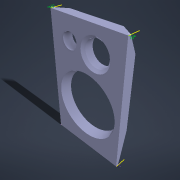
# Autodesk Inventor part: Front
Saved by Autodesk Inventor 2022 (Build 260153000, 153)
## iProperties
Created: 2022-03-29
Part Number: Front
Material: Пластик АБС
Document SubType Name: Modeling
Designer: Kalugin_a
Density: 1.06 g/cm^3
Appearance: Грифельно-синий
Author: Kalugin_a
Autodesk Inventor part; units mm, degrees
ref_plane "YZ Plane" through (0, 0, 0) normal (1, 0, 0) x (0, 1, 0)
ref_plane "XZ Plane" through (0, 0, 0) normal (0, 1, 0) x (-1, 0, 0)
ref_plane "XY Plane" through (0, 0, 0) normal (0, 0, 1) x (1, 0, 0)
sketch "Эскиз1" plane through (0, 0, 0) normal (0, 0, 1) x (1, 0, 0)
  line L0 (0, 0) -> (290, 0)
  line L1 (290, 0) -> (290, 470)
  line L2 (290, 470) -> (0, 470)
  line L3 (0, 470) -> (0, 0)
  line L4 (145, 470) -> (145, 0) construction
  circle A0 centre (145, 180) radius 133
  circle A1 centre (145, 180) radius 115
  circle A2 centre (80, 390) radius 47
  circle A3 centre (80, 390) radius 30
  line L5 (136.9264, 433.5) -> (229.9264, 433.5)
  line L6 (236.9264, 426.5) -> (236.9264, 333.5)
  line L7 (229.9264, 326.5) -> (136.9264, 326.5)
  line L8 (129.9264, 333.5) -> (129.9264, 426.5)
  line L9 (129.9264, 433.5) -> (236.9264, 326.5) construction
  line L10 (236.9264, 433.5) -> (129.9264, 326.5) construction
  circle A4 centre (183.4264, 380) radius 47
  circle A5 centre (183.4264, 380) radius 58 construction
  line L11 (0, 160) -> (60, 0)
  line L12 (290, 160) -> (230, 0)
  line L13 (50, 470) -> (0, 400)
  line L14 (240, 470) -> (290, 400)
  line L15 (290, 320) -> (0, 320) construction
  arc A6 (236.9264, 429.5) -> (232.9264, 433.5) centre (232.9264, 429.5) ccw
  arc A7 (236.9264, 426.5) -> (229.9264, 433.5) centre (229.9264, 426.5) ccw
  arc A8 (136.9264, 433.5) -> (129.9264, 426.5) centre (136.9264, 426.5) ccw
  arc A9 (129.9264, 333.5) -> (136.9264, 326.5) centre (136.9264, 333.5) ccw
  arc A10 (229.9264, 326.5) -> (236.9264, 333.5) centre (229.9264, 333.5) ccw
  line L16 (0, 320) -> (290, 320)
  dimension "d0" = 290
  dimension "d1" = 470
  dimension "d3" = 266
  dimension "d4" = 230
  dimension "d5" = 94
  dimension "d6" = 60
  dimension "d9" = 94
  dimension "d11" = 380
  dimension "d12" = 390
  dimension "d13" = 180
  dimension "d14" = 160
  dimension "d15" = 60
  dimension "d16" = 160
  dimension "d17" = 60
  dimension "d18" = 50
  dimension "d19" = 70
  dimension "d20" = 80
  dimension "d21" = 50
  dimension "d38" = 70
  dimension "d39" = 320
  dimension "d47" = 4
  dimension "d48" = 7
  constraints: 34 end point, 20 point on line, 11 centre point, 10 point on circle, 10 tangent, 5 equal length, 4 perpendicular, 3 coincident, 3 equal radius, 3 horizontal, 3 midpoint
  measures "d0" distance of L2.end L1.end
  measures "d1" distance of L1.end L0.end
  measures "d3" diameter of A0
  measures "d4" diameter of A1
  measures "d5" diameter of A2
  measures "d6" diameter of A3
  measures "d9" diameter of A4
  measures "d11" distance from line of L0 A5.centre
  measures "d12" distance from line of L0 A2.centre
  measures "d13" distance of L4.end A0.centre
  measures "d14" distance of L0.start L11.start
  measures "d15" distance of L0.start L11.end
  measures "d16" distance of L0.end L12.start
  measures "d17" distance of L0.end L12.end
  measures "d18" distance of L2.end L13.start
  measures "d19" distance of L2.end L13.end
  measures "d20" distance from line of L3 A2.centre
  measures "d21" distance of L1.end L14.start
  measures "d38" distance of L1.end L14.end
  measures "d39" distance between parallel lines of L0 L15
  measures "d47" radius of A6
  measures "d48" radius of A7
extrude "Выдавливание1" add sketch "Эскиз1" along normal blind 42 contours L3 L11 L0 | L11 L3 L16 L1 L12 L0 | L12 L1 L0 | L3 L13 L2 L14 L1 L16 | L3 L2 L13 | L14 L2 L1 | A0 | A2 | L5 A7 L6 A10 L7 A9 L8 A8
sketch "Эскиз3" plane through (0, 470, 0) normal (0, 1, 0) x (1, 0, 0)
  line L0 (290, 0) -> (290, -42) projected
  line L1 (0, 0) -> (0, -42) projected
  point P0 (290, -32)
  point P1 (0, -32)
  dimension "d24" = 10
  dimension "d25" = 10
  constraints: 2 point on line
  measures "d24" distance of L0.end point (290, -32)
  measures "d25" distance of L1.end point (0, -32)
sketch "Эскиз4" plane through (0, 0, 0) normal (0, -1, 0) x (1, 0, 0)
  line L0 (0, 0) -> (0, 42) projected
  line L1 (290, 0) -> (290, 42) projected
  point P0 (0, 32)
  point P1 (290, 32)
  constraints: 2 point on line
chamfer "Фаска2" distance 10 distance2 30 1 edges at (30, 180, 42) measured on face at (29.5, 180, 42)
chamfer "Фаска3" distance 10 angle 45 1 edges at (136.4264, 380, 42)
ref_plane "РабПлоскость8" through (0, 470, 32) normal (-0.5030521, 0.3593229, -0.7860189) x (0.8422714, 0, -0.5390537)
split "Разделение8" plane through (0, 470, 32) removes the side toward (-0.5030521, 0.3593229, -0.7860189)
ref_plane "РабПлоскость9" through (290, 470, 32) normal (-0.5030521, -0.3593229, 0.7860189) x (-0.8422714, 0, -0.5390537)
split "Разделение9" plane through (290, 470, 32) removes the side toward (0.5030521, 0.3593229, -0.7860189)
ref_plane "РабПлоскость10" through (0, 0, 32) normal (0.4634276, 0.1737853, 0.8689267) x (0.8823529, 0, -0.4705882)
split "Разделение10" plane through (0, 0, 32) removes the side toward (-0.4634276, -0.1737853, -0.8689267)
ref_plane "РабПлоскость11" through (290, 0, 32) normal (-0.4634276, 0.1737853, 0.8689267) x (0, 0.9805807, -0.1961161)
split "Разделение11" plane through (290, 0, 32) removes the side toward (0.4634276, -0.1737853, -0.8689267)
chamfer "Фаска5" distance 4 angle 45 4 edges at (290, 280, 0) (145, 470, 0) (0, 280, 0) (145, 0, 0)
extrude "Выдавливание2" cut sketch "Эскиз1" along normal blind 4 contours A0 | A1
extrude "Выдавливание3" cut sketch "Эскиз1" along normal blind 4 contours A2
extrude "Выдавливание4" cut sketch "Эскиз1" along normal blind 2 contours L5 A7 L6 A10 L7 A9 L8 A8
